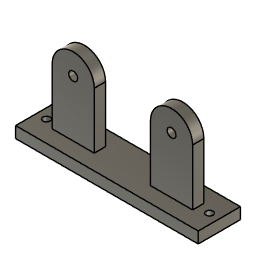
rod supporter v6 (Autodesk Fusion 360 design; units mm, degrees)
Autodesk Fusion 360 part; units mm, degrees
sketch "草图1" plane through (0, 0, 0) normal (0, 0, 1) x (1, 0, 0)
  line L0 (-65, 15) -> (65, 15)
  line L1 (65, 15) -> (65, -15)
  line L2 (65, -15) -> (-65, -15)
  line L3 (-65, -15) -> (-65, 15)
  line L4 (1.75, 0) -> (22.5, 0)
  line L5 (0, 1.75) -> (0, 22.5)
  circle A0 centre (58, 0) radius 2.5
  circle A1 centre (-58, 0) radius 2.5
  dimension "d1" = 130
  dimension "d2" = 30
  dimension "d16" = 5
  dimension "d17" = 58
  dimension "d18" = 5
  constraint horizontal L0
  constraint perpendicular L0 L1
  constraint perpendicular L1 L2
  constraint perpendicular L0 L3
  constraint symmetric L0 L2 L4
  constraint symmetric L1 L3 L5
  constraint symmetric L5 A0.centre A1.centre
  constraint horizontal origin A0.centre
  measures "d1" distance of L0.start L0.end
  measures "d2" distance of L0.end L1.end
  measures "d16" diameter of A0
  measures "d17" distance of origin A0.centre
  measures "d18" diameter of A1
extrude "拉伸1" add sketch "草图1" against normal blind 8
ref_plane "工作平面1" through (0, 4, 0) normal (0, 1, 0) x (0, 0, 1)
sketch "草图2" plane through (0, 4, 0) normal (0, 1, 0) x (1, 0, 0)
  line L0 (50, 0) -> (20, 0)
  line L1 (20, 0) -> (20, -40)
  line L2 (20, -40) -> (50, -40)
  line L3 (50, -40) -> (50, 0)
  circle A0 centre (35, -40) radius 15
  circle A1 centre (35, -40) radius 3.175
  dimension "d6" = 30
  dimension "d7" = 40
  dimension "d8" = 20
  dimension "d9" = 6.35
  dimension "d14" = 35
  dimension "d15" = 35
  constraint horizontal L0
  constraint perpendicular L0 L1
  constraint perpendicular L1 L2
  constraint perpendicular L0 L3
  constraint horizontal origin L0.end
  constraint coincident L1.end A0
  constraint horizontal L2.end A0.centre
  measures "d6" distance of L0.start L0.end
  measures "d7" distance of L0.start L2.end
  measures "d8" distance of origin L0.end
  measures "d9" diameter of A1
  measures "d14" horizontal distance of origin A0.centre
  measures "d15" horizontal distance of origin A0.centre
extrude "拉伸2" add sketch "草图2" against normal blind 8 contours L0 L1 L3 A0 | L2 A0 A1 | L2 A0 A1
mirror "镜像1" about plane through (0, 0, 0) normal (1, 0, 0) of bodies 1 merged
equation "d18 = d16"
